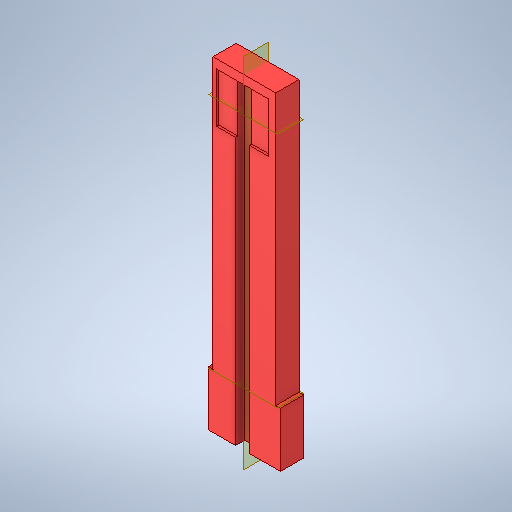
# Autodesk Inventor part: Halter_PP
Saved by Autodesk Inventor 2025 (Build 290162000, 162)
## iProperties
Created: 2018-10-16
Part Number: Halter_PP
Material: ABS-Kunststoff
Document SubType Name: Modeling
Designer: LK-Desktop
Density: 1.06 g/cm^3
Appearance: Glatt - Weiß
Kerbentiefe: 0,000 mm
b_Halter: 13,500 mm
Kerbenbreite: 1,200 mm
d_Halter: 5,000 mm
Author: LK-Desktop
Autodesk Inventor part; units mm, degrees
ref_plane "YZ Plane" through (0, 0, 0) normal (1, 0, 0) x (0, 1, 0)
ref_plane "XZ Plane" through (0, 0, 0) normal (0, 1, 0) x (-1, 0, 0)
ref_plane "XY Plane" through (0, 0, 0) normal (0, 0, 1) x (1, 0, 0)
sketch "Skizze4" plane through (0, 0, 0) normal (0, 1, 0) x (-1, 0, 0)
  line L0 (-33.6472, -5.1972) -> (-47.1472, -5.1972)
  line L1 (-47.1472, -5.1972) -> (-47.1472, -7.0972)
  line L2 (-47.1472, -7.0972) -> (-47.1472, -7.0972)
  line L3 (-47.1472, -7.0972) -> (-47.1472, -8.2972)
  line L4 (-47.1472, -8.2972) -> (-47.1472, -8.2972)
  line L5 (-47.1472, -8.2972) -> (-47.1472, -10.1972)
  line L6 (-47.1472, -10.1972) -> (-33.6472, -10.1972)
  line L7 (-33.6472, -10.1972) -> (-33.6472, -8.2972)
  line L8 (-33.6472, -8.2972) -> (-33.6472, -8.2972)
  line L9 (-33.6472, -8.2972) -> (-33.6472, -7.0972)
  line L10 (-33.6472, -7.0972) -> (-33.6472, -7.0972)
  line L11 (-33.6472, -7.0972) -> (-33.6472, -5.1972)
  dimension "Kerbentiefe" = 0
  dimension "b_Halter" = 13.5
  dimension "d12" = 0
  dimension "Kerbenbreite" = 1.2
  dimension "d_Halter" = 5
  constraints: 24 end point, 7 perpendicular, 4 collinear, 3 point on line, 2 equal length, 1 horizontal
  measures "Kerbentiefe" distance of L3.end L4.end
  measures "b_Halter" distance of L5.end L6.end
  measures "d12" distance of L7.end L8.end
  measures "Kerbenbreite" distance of L8.end L9.end
  measures "d_Halter" distance between parallel lines of L6 L0
extrude "Extrusion3" add sketch "Skizze4" along normal blind 70
sketch "Skizze6" plane through (33.6472, 0, -5.1972) normal (0, 0, 1) x (1, 0, 0)
  line L0 (0, 70) -> (13.5, 70) projected
  line L1 (0.75, 68.1) -> (11.95, 68.1)
  line L2 (11.95, 68.1) -> (11.95, 57.4)
  line L3 (11.95, 57.4) -> (0.75, 57.4)
  line L4 (0.75, 57.4) -> (0.75, 68.1)
  line L5 (0, 0) -> (13.5, 0) projected
  line L6 (6.75, 70) -> (6.75, 0) construction
  dimension "d20" = 1.9
  dimension "d21" = 10.7
  dimension "d22" = 11.2
  dimension "d31" = 5.2
  constraints: 10 end point, 3 perpendicular, 2 midpoint
  measures "d20" distance between parallel lines of L0 L1
  measures "d21" distance of L1.end L2.end
  measures "d22" distance of L2.end L3.end
  measures "d31" distance between parallel lines of L2 L6
extrude "Extrusion5" cut sketch "Skizze6" against normal blind 0.5
sketch "Skizze7" plane through (33.6472, 0, -5.1972) normal (0, 0, 1) x (1, 0, 0)
  line L0 (0.75, 68.1) -> (11.95, 68.1) projected
  line L1 (0, 0) -> (13.5, 0) projected
  line L2 (0.75, 68.1) -> (11.95, 68.1) projected
  line L3 (4.85, 68.1) -> (7.85, 68.1)
  line L4 (7.85, 68.1) -> (7.85, 0)
  line L5 (7.85, 0) -> (4.85, 0)
  line L6 (4.85, 0) -> (4.85, 68.1)
  line L7 (0.75, 57.4) -> (0.75, 68.1) projected
  dimension "d26" = 3
  dimension "d32" = 4.1
  constraints: 8 end point, 5 point on line
  measures "d26" distance between parallel lines of L4 L6
  measures "d32" distance between parallel lines of L7 L6
extrude "Extrusion6" cut sketch "Skizze7" against normal blind 2
ref_plane "hor_Strahlebene" through (34.3972, 62.75, -5.1972) normal (0, 1, 0) x (1, 0, 0)
ref_plane "Ebene_Anschlag2" through (34.3972, 11.75, -5.1972) normal (0, 1, 0) x (1, 0, 0)
sketch "Skizze10" plane through (0, 0, 0) normal (0, -1, 0) x (1, 0, 0)
  line L0 (33.6472, -5.1972) -> (32.6472, -5.1972)
  line L1 (32.6472, -5.1972) -> (32.6472, -10.1972)
  line L2 (32.6472, -10.1972) -> (33.6472, -10.1972)
  line L3 (33.6472, -10.1972) -> (33.6472, -5.1972)
  dimension "d36" = 1
  constraints: 8 end point
  measures "d36" distance of L2.end L1.end
extrude "Extrusion8" add sketch "Skizze10" against normal up to surface (11.75 mm away)
ref_plane "Mittelebene_Halter" through (40.3972, 70, -10.1972) normal (-1, 0, 0) x (0, 0, 1)
mirror "Spiegeln1" about plane through (40.3972, 70, -10.1972) normal (-1, 0, 0) of "Extrusion8"
ref_plane "Arbeitsebene4" through (40.3972, 70, -10.1972) normal (-1, 0, 0) x (0, 0, 1)
equation "\"d32\" = -0.5 * d26 + 0.5 * d22"
